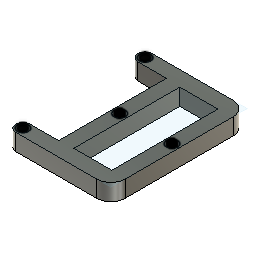
goon v1 (Autodesk Fusion 360 design; units mm, degrees)
Autodesk Fusion 360 part; units mm, degrees
note: some values were not read from the file. Set by a fixed rule: which sketch regions a step uses.
sketch "Sketch1" plane through (0, 0, 0) normal (0, 0, 1) x (1, 0, 0)
  line L0 (10, 27.85) -> (-10, 27.85)
  line L1 (-10, 27.85) -> (-10, -27.85)
  line L2 (-10, -27.85) -> (10, -27.85)
  line L3 (10, -27.85) -> (10, 27.85)
  line L4 (10, 27.85) -> (-10, -27.85) construction
  line L5 (-10, 27.85) -> (10, -27.85) construction
  line L6 (-10, 0) -> (-17.5, 0) construction
  line L7 (10, 0) -> (17.5, 0) construction
  line L8 (0, 27.85) -> (0, 35.85) construction
  line L9 (0, -27.85) -> (0, -35.85) construction
  line L10 (17.5, 0) -> (17.5, 35.85)
  line L11 (0, 35.85) -> (17.5, 35.85)
  line L12 (17.5, 35.85) -> (-17.5, 35.85)
  line L13 (-17.5, 35.85) -> (-17.5, -35.85)
  line L14 (-17.5, -35.85) -> (17.5, -35.85)
  line L15 (17.5, -35.85) -> (17.5, 35.85)
  line L16 (-17.5, 35.85) -> (-32.5, 35.85)
  line L17 (-32.5, 35.85) -> (-32.5, 28.35)
  line L18 (-32.5, 28.35) -> (-17.5, 28.35)
  line L19 (-17.5, -35.85) -> (-32.5, -35.85)
  line L20 (-32.5, -35.85) -> (-32.5, -28.35)
  line L21 (-32.5, -28.35) -> (-17.5, -28.35)
  circle A0 centre (-32.5, 32.1) radius 3.75
  circle A1 centre (-32.5, -32.1) radius 3.75
  dimension "d1" = 20
  dimension "d2" = 55.7
  dimension "d3" = 7.5
  dimension "d4" = 7.5
  dimension "d5" = 8
  dimension "d6" = 8
  dimension "d7" = 35
  dimension "d8" = 15
  dimension "d9" = 7.5
  dimension "d10" = 15
  dimension "d11" = 7.5
  constraint horizontal L0
  constraint perpendicular L0 L1
  constraint parallel L0 L2
  constraint parallel L1 L3
  constraint coincident L4 origin
  constraint coincident L5 origin
  constraint midpoint L1 L6.start
  constraint perpendicular L1 L6
  constraint midpoint L3 L7.start
  constraint perpendicular L3 L7
  constraint midpoint L0 L8.start
  constraint perpendicular L0 L8
  constraint midpoint L2 L9.start
  constraint perpendicular L2 L9
  constraint horizontal L12
  constraint vertical L13
  constraint horizontal L14
  constraint vertical L15
  constraint perpendicular L13 L16
  constraint perpendicular L12 L17
  constraint coincident L13 L18.end
  constraint perpendicular L13 L18
  constraint perpendicular L13 L19
  constraint perpendicular L19 L20
  constraint coincident L13 L21.end
  constraint perpendicular L13 L21
  constraint midpoint L17 A0.centre
  constraint coincident L16.end A0
  constraint midpoint L20 A1.centre
  constraint coincident L20.end A1
  measures "d1" distance of L1.end L2.end
  measures "d2" distance of L0.end L1.end
  measures "d3" distance of L6.start L6.end
  measures "d4" distance of L7.start L7.end
  measures "d5" distance of L8.start L8.end
  measures "d6" distance of L9.start L9.end
  measures "d7" distance of L10.end L12.end
  measures "d8" distance of L12.end L16.end
  measures "d9" distance of L16.end L17.end
  measures "d10" distance of L13.end L19.end
  measures "d11" distance of L19.end L20.end
extrude "Extrude1" add sketch "Sketch1" along normal blind 8.75
sketch "Sketch2" plane through (0, 0, 8.75) normal (0, 0, 1) x (-1, 0, 0)
  line L0 (-10, -27.85) -> (-10, 27.85)
  line L1 (-10, 27.85) -> (10, 27.85)
  line L2 (10, 27.85) -> (10, -27.85)
  line L3 (10, -27.85) -> (-10, -27.85)
  line L4 (32.5, 35.85) -> (-17.5, 35.85)
  line L5 (-17.5, 35.85) -> (-17.5, -35.85)
  line L6 (-17.5, -35.85) -> (32.5, -35.85)
  arc A0 (32.5, -35.85) -> (32.5, -28.35) centre (32.5, -32.1) ccw
  line L7 (32.5, -28.35) -> (17.5, -28.35)
  line L8 (17.5, -28.35) -> (17.5, 28.35)
  line L9 (17.5, 28.35) -> (32.5, 28.35)
  arc A1 (32.5, 28.35) -> (32.5, 35.85) centre (32.5, 32.1) ccw
  circle A2 centre (32.5, -32.1) radius 2.925
  circle A3 centre (32.5, 32.1) radius 2.925
  circle A4 centre (32.5, -32.1) radius 1.875
  circle A5 centre (32.5, 32.1) radius 1.875
  line L10 (17.5, 0) -> (10, 0) construction
  line L11 (-10, 0) -> (-17.5, 0) construction
  circle A6 centre (13.75, 0) radius 2.925
  circle A7 centre (13.75, 0) radius 1.875
  circle A8 centre (-13.75, 0) radius 2.925
  circle A9 centre (-13.75, 0) radius 1.875
  dimension "d14" = 5.85
  dimension "d15" = 5.85
  dimension "d16" = 3.75
  dimension "d17" = 3.75
  dimension "d18" = 5.85
  dimension "d19" = 3.75
  dimension "d20" = 5.85
  dimension "d21" = 3.75
  constraint concentric A0 A2
  constraint concentric A1 A3
  constraint concentric A2 A4
  constraint concentric A3 A5
  constraint midpoint L8 L10.start
  constraint midpoint L2 L10.end
  constraint midpoint L0 L11.start
  constraint midpoint L5 L11.end
  constraint midpoint L10 A6.centre
  constraint concentric A6 A7
  constraint midpoint L11 A8.centre
  constraint concentric A8 A9
  measures "d14" diameter of A2
  measures "d15" diameter of A3
  measures "d16" diameter of A4
  measures "d17" diameter of A5
  measures "d18" diameter of A6
  measures "d19" diameter of A7
  measures "d20" diameter of A8
  measures "d21" diameter of A9
extrude "Extrude2" cut sketch "Sketch2" against normal blind 26 contours A4 | A5 | A7 | A9
extrude "Extrude3" cut sketch "Sketch2" against normal blind 3.1 contours A2 | A3 | A6 | A8
fillet "Fillet1" radius 7.5 2 edges at (17.5, 35.85, 4.375) (17.5, -35.85, 4.375)
